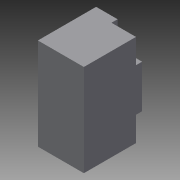
# Autodesk Inventor part: Baterie
Saved by Autodesk Inventor 2018.2 (Build 222227000, 227)
## iProperties
Created: 2019-03-20
Part Number: Baterie
Material: Generisch
Document SubType Name: Modeling
Designer: Lolob
Density: 1 g/cm^3
Appearance: Vorgabe
Author: Lolob
Autodesk Inventor part; units mm, degrees
ref_plane "YZ Plane" through (0, 0, 0) normal (1, 0, 0) x (0, 1, 0)
ref_plane "XZ Plane" through (0, 0, 0) normal (0, 1, 0) x (-1, 0, 0)
ref_plane "XY Plane" through (0, 0, 0) normal (0, 0, 1) x (1, 0, 0)
sketch "Skizze1" plane through (0, 0, 0) normal (0, 1, 0) x (-1, 0, 0)
  line L0 (159.3398, 191.458) -> (9.3398, 191.458)
  line L1 (9.3398, 191.458) -> (9.3398, -108.542)
  line L2 (9.3398, -108.542) -> (159.3398, -108.542)
  line L3 (159.3398, -108.542) -> (159.3398, 191.458)
  point P0 (0, 0)
  dimension "d0" = 300
  dimension "d1" = 150
  constraints: 8 end point, 2 parallel, 1 horizontal, 1 perpendicular
  measures "d0" distance of L2.end L0.start
  measures "d1" distance of L0.start L0.end
extrude "Extrusion1" add sketch "Skizze1" along normal blind 190
sketch "Skizze2" plane through (0, 190, 0) normal (0, 1, 0) x (1, 0, 0)
  line L0 (-9.3398, 108.542) -> (-159.3398, 108.542) projected
  line L1 (-159.3398, -191.458) -> (-9.3398, -191.458) projected
  line L2 (-9.3398, -191.458) -> (-9.3398, 108.542) projected
  line L3 (-9.3398, 108.542) -> (-159.3398, 108.542) projected
  line L4 (-159.3398, 108.542) -> (-159.3398, -191.458) projected
  line L5 (-9.3398, 108.542) -> (-89.3398, 108.542)
  line L6 (-89.3398, 108.542) -> (-89.3398, 48.542)
  line L7 (-69.3398, 28.542) -> (-9.3398, 28.542)
  line L8 (-9.3398, 28.542) -> (-9.3398, 108.542)
  line L9 (-9.3398, -191.458) -> (-9.3398, 108.542) projected
  line L10 (-9.3398, -191.458) -> (-89.3398, -191.458)
  line L11 (-89.3398, -191.458) -> (-89.3398, -131.458)
  line L12 (-69.3398, -111.458) -> (-9.3398, -111.458)
  line L13 (-9.3398, -111.458) -> (-9.3398, -191.458)
  arc A0 (-69.3398, -111.458) -> (-89.3398, -131.458) centre (-69.3398, -131.458) ccw
  arc A1 (-89.3398, 48.542) -> (-69.3398, 28.542) centre (-69.3398, 48.542) ccw
  point P0 (0, 0)
  point P1 (-89.3398, 28.542)
  point P2 (-89.3398, -111.458)
  dimension "d4" = 80
  dimension "d5" = 80
  dimension "d6" = 80
  dimension "d7" = 80
  dimension "d8" = 20
  dimension "d9" = 20
  constraints: 16 end point, 4 parallel, 4 point on circle, 4 point on line, 4 tangent, 2 centre point, 2 horizontal, 2 perpendicular
  measures "d4" distance of L7.end point (-89.34, 28.542)
  measures "d5" distance of point (-89.34, 28.542) L5.end
  measures "d6" distance of point (-89.34, -111.458) L12.end
  measures "d7" distance of L10.end point (-89.34, -111.458)
  measures "d8" radius of A0
  measures "d9" radius of A1
extrude "Extrusion2" cut sketch "Skizze2" against normal blind 20 contours L2 L7 A1 L6 L0 | L2 L1 L11 A0 L12
sketch "Skizze3" plane through (0, 170, 0) normal (0, 1, 0) x (1, 0, 0)
  line L0 (-9.3398, -111.458) -> (-9.3398, -191.458) projected
  line L1 (-69.3398, -111.458) -> (-9.3398, -111.458) projected
  arc A0 (-69.3398, -111.458) -> (-89.3398, -131.458) centre (-69.3398, -131.458) ccw projected
  line L2 (-89.3398, -191.458) -> (-89.3398, -131.458) projected
  line L3 (-9.3398, -191.458) -> (-89.3398, -191.458) projected
  line L4 (-9.3398, 108.542) -> (-9.3398, 28.542) projected
  line L5 (-89.3398, 108.542) -> (-9.3398, 108.542) projected
  line L6 (-89.3398, 48.542) -> (-89.3398, 108.542) projected
  arc A1 (-89.3398, 48.542) -> (-69.3398, 28.542) centre (-69.3398, 48.542) ccw projected
  line L7 (-9.3398, 28.542) -> (-69.3398, 28.542) projected
  circle A2 centre (-49.3398, -151.458) radius 7.5
  circle A3 centre (-49.3398, 68.542) radius 7.5
  point P0 (0, 0)
  dimension "d12" = 15
  dimension "d13" = 15
  dimension "d16" = 40
  dimension "d17" = 40
  dimension "d18" = 40
  dimension "d19" = 40
  constraints: 2 centre point
  measures "d12" diameter of A2
  measures "d13" diameter of A3
  measures "d16" distance from line of L7 A3.centre
  measures "d17" distance from line of L4 A3.centre
  measures "d18" distance from line of L0 A2.centre
  measures "d19" distance from line of L3 A2.centre
extrude "Extrusion3" add sketch "Skizze3" along normal blind 20 contours A2 | A3
